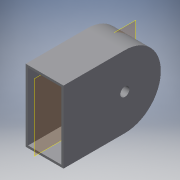
# Autodesk Inventor part: EncoderEnclosure
Saved by Autodesk Inventor 2018.3 (Build 223284000, 284)
## iProperties
Created: 2018-06-30
Part Number: EncoderEnclosure
Material: Generisch
Document SubType Name: Modeling
Designer: JochenAlt
Density: 1 g/cm^3
Appearance: Vorgabe
Author: JochenAlt
Autodesk Inventor part; units mm, degrees
ref_plane "YZ Plane" through (0, 0, 0) normal (1, 0, 0) x (0, 1, 0)
ref_plane "XZ Plane" through (0, 0, 0) normal (0, 1, 0) x (-1, 0, 0)
ref_plane "XY Plane" through (0, 0, 0) normal (0, 0, 1) x (1, 0, 0)
ref_plane "Arbeitsebene1" through (0, 0, 0) normal (1, 0, 0) x (0, 0, -1)
sketch "Skizze1" plane through (0, 0, 0) normal (1, 0, 0) x (0, 0, -1)
  arc A0 (15.7, 0) -> (-15.7, 0) centre (0, 0) ccw
  line L0 (15.7, 0) -> (15.7, -26.8)
  line L1 (15.7, -26.8) -> (-15.7, -26.8)
  line L2 (-15.7, -26.8) -> (-15.7, 0)
  circle A1 centre (0, 0) radius 2
  point P0 (0, 15.7)
  dimension "d0" = 31.4
  dimension "d1" = 42.5
  dimension "d2" = 4
  constraints: 6 end point, 3 point on circle, 2 centre point, 2 coincident, 1 parallel
  measures "d0" distance of L0.end L1.end
  measures "d1" distance from line of L1 point (0, 15.7)
  measures "d2" diameter of A1
extrude "Extrusion1" add sketch "Skizze1" along normal blind 10 and the other way blind 6.5
shell "Wandung1" thickness 1 removed faces 1 at (-1, -26.8, -5.2333)
